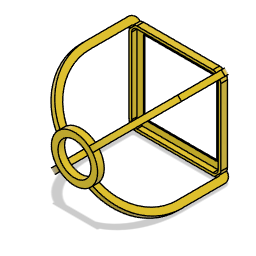
Livox Protection (Autodesk Fusion 360 design; units mm, degrees)
Autodesk Fusion 360 part; units mm, degrees
note: some values were not read from the file. Set by a fixed rule: which sketch regions a step uses.
sketch "Sketch1" plane through (0, 0, 0) normal (0, 0, 1) x (1, 0, 0)
  line L0 (28.75, 32.75) -> (-28.75, 32.75)
  line L1 (-32.75, 28.75) -> (-32.75, -28.75)
  line L2 (-28.75, -32.75) -> (28.75, -32.75)
  line L3 (32.75, -28.75) -> (32.75, 28.75)
  line L4 (32.75, 32.75) -> (-32.75, -32.75) construction
  line L5 (-32.75, 32.75) -> (32.75, -32.75) construction
  arc A0 (-28.75, 32.75) -> (-32.75, 28.75) centre (-28.75, 28.75) ccw
  arc A1 (32.75, 28.75) -> (28.75, 32.75) centre (28.75, 28.75) ccw
  arc A2 (28.75, -32.75) -> (32.75, -28.75) centre (28.75, -28.75) ccw
  arc A3 (-32.75, -28.75) -> (-28.75, -32.75) centre (-28.75, -28.75) ccw
  line L6 (-34.75, 28.75) -> (-34.75, -28.75)
  arc A4 (-34.75, -28.75) -> (-28.75, -34.75) centre (-28.75, -28.75) ccw
  line L7 (-28.75, -34.75) -> (28.75, -34.75)
  arc A5 (28.75, -34.75) -> (34.75, -28.75) centre (28.75, -28.75) ccw
  line L8 (34.75, -28.75) -> (34.75, 28.75)
  arc A6 (34.75, 28.75) -> (28.75, 34.75) centre (28.75, 28.75) ccw
  line L9 (28.75, 34.75) -> (-28.75, 34.75)
  arc A7 (-28.75, 34.75) -> (-34.75, 28.75) centre (-28.75, 28.75) ccw
  line L10 (-27.75, 27.75) -> (-27.75, -27.75)
  line L11 (-27.75, -27.75) -> (27.75, -27.75)
  line L12 (27.75, -27.75) -> (27.75, 27.75)
  line L13 (27.75, 27.75) -> (-27.75, 27.75)
  dimension "d1" = 65.5
  dimension "d2" = 65.5
  dimension "d3" = 4
  dimension "d4" = 4
  dimension "d5" = 4
  dimension "d6" = 4
  dimension "d7" = 2
  dimension "d8" = -5
  constraint horizontal L0
  constraint perpendicular L0 L1
  constraint parallel L0 L2
  constraint parallel L1 L3
  constraint coincident L4 origin
  constraint coincident L5 origin
  constraint coincident L5.start L0
  constraint coincident L5.start L1
  constraint tangent L0 A0
  constraint tangent L1 A0
  constraint coincident L4.start L0
  constraint coincident L4.start L3
  constraint tangent L0 A1
  constraint tangent L3 A1
  constraint coincident L5.end L2
  constraint coincident L5.end L3
  constraint tangent L2 A2
  constraint tangent L3 A2
  constraint coincident L4.end L2
  constraint coincident L4.end L1
  constraint tangent L2 A3
  constraint tangent L1 A3
  measures "d1" distance of L4.start L5.start
  measures "d2" distance of L4.start L5.end
  measures "d3" radius of A0
  measures "d4" radius of A1
  measures "d5" radius of A2
  measures "d6" radius of A3
extrude "Extrude1" add sketch "Sketch1" along normal blind 1 contours L0 L1 L2 L3 A0 A1 A2 A3 makes body 1
extrude "Extrude2" add sketch "Sketch1" along normal blind 5 contours L6 A4 L7 A5 L8 A6 L9 A7 bodies 1
ref_plane "WorkPlane1" through (0, 0, 76) normal (0, 0, 1) x (1, 0, 0)
sketch "Sketch2" plane through (0, 0, 76) normal (0, 0, 1) x (1, 0, 0)
  circle A0 centre (0, 0) radius 12.5
  line L0 (-27.75, 27.75) -> (27.75, 27.75)
  line L1 (27.75, 27.75) -> (27.75, -27.75)
  line L2 (27.75, -27.75) -> (-27.75, -27.75)
  line L3 (-27.75, -27.75) -> (-27.75, 27.75)
  arc A1 (-32.75, -28.75) -> (-28.75, -32.75) centre (-28.75, -28.75) ccw
  line L4 (-28.75, -32.75) -> (28.75, -32.75)
  arc A2 (28.75, -32.75) -> (32.75, -28.75) centre (28.75, -28.75) ccw
  line L5 (32.75, -28.75) -> (32.75, 28.75)
  arc A3 (32.75, 28.75) -> (28.75, 32.75) centre (28.75, 28.75) ccw
  line L6 (28.75, 32.75) -> (-28.75, 32.75)
  arc A4 (-28.75, 32.75) -> (-32.75, 28.75) centre (-28.75, 28.75) ccw
  line L7 (-32.75, 28.75) -> (-32.75, -28.75)
  line L8 (-27.75, -27.75) -> (27.75, -27.75)
  line L9 (32.75, 32.75) -> (-32.75, -32.75)
  circle A5 centre (0, 0) radius 17.5
  dimension "d14" = 25
  dimension "d27" = 17.5
  constraint coincident A0.centre A5.centre
  measures "d14" diameter of A0
  measures "d27" radius of A5
extrude "Extrude3" add sketch "Sketch2" along normal blind 5 separate body contours A0 L9 A5 | A0 L9 A5 makes body 2
ref_plane "WorkPlane2" through (0, 0, 0) normal (0.707107, -0.707107, 0) x (0.707107, 0.707107, 0)
sketch "Sketch3" plane through (0, 0, 0) normal (0.707107, -0.707107, 0) x (0.707107, 0.707107, 0)
  line L0 (46.6586, 0) -> (44.9013, 0)
  line L1 (44.9013, 0) -> (44.9013, 5)
  line L2 (46.6586, 5) -> (44.9013, 5)
  line L3 (44.9013, 5) -> (44.9013, 0)
  line L4 (17.5, 81) -> (17.5, 76)
  line L5 (17.5, 81) -> (-17.5, 81)
  line L6 (17.5, 76) -> (-17.5, 76)
  line L7 (0, 0) -> (0, 76) construction
  line L8 (-78.4678, 38) -> (78.4678, 38) construction
  line L9 (46.6586, 5) -> (46.6586, 38)
  line L10 (46.6586, 0) -> (51.6586, 0)
  line L11 (51.6586, 0) -> (51.6586, 38)
  arc A0 (46.6586, 38) -> (17.5, 76) centre (7.3182, 38) ccw
  arc A1 (51.6586, 38) -> (17.5, 81) centre (7.5144, 38) ccw
  dimension "d29" = 5
  constraint coincident L4.end L6.start
  constraint coincident L7.start origin
  constraint midpoint L6 L7.end
  constraint perpendicular L7 L8
  constraint midpoint L7 L8
  constraint coincident L2.start L9.start
  constraint coincident L8 L9.end
  constraint perpendicular L8 L9
  constraint coincident L0.start L10.start
  constraint perpendicular L9 L10
  constraint coincident L8 L11.end
  constraint perpendicular L8 L11
  constraint coincident L4.start L5.start
  constraint tangent L9 A0
  constraint tangent L11 A1
  measures "d29" distance of L9 L11
extrude "Extrude4" add sketch "Sketch3" along normal mid plane 4 bodies 1 2
mirror "Mirror1" about plane through (0, 0, 0) normal (1, 0, 0) of "Extrude4"
mirror "Mirror2" about plane through (0, 0, 0) normal (0, 1, 0) of "Extrude4", "Mirror1"
fillet "Fillet1" radius 5 4 edges at (36.5282, 36.5282, 0) (36.5282, -36.5282, 0) (-36.5282, 36.5282, 0) (-36.5282, -36.5282, 0) on bodies 1
fillet "Fillet1" radius 1 4 edges at (32.9926, 32.9926, 5) (-32.9926, 32.9926, 5) (-32.9926, -32.9926, 5) (32.9926, -32.9926, 5) on bodies 1
